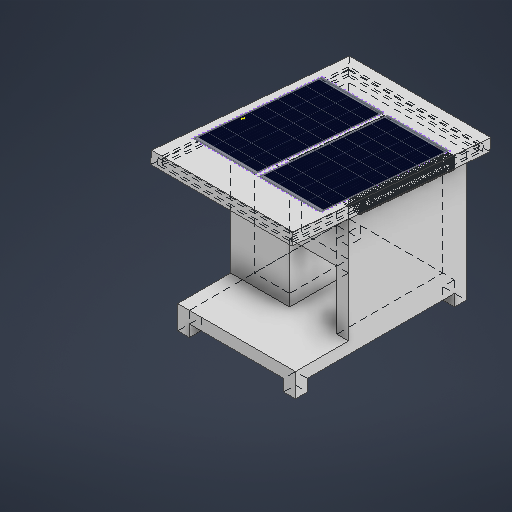
# Autodesk Inventor part: Cat House
Saved by Autodesk Inventor 2026 (Build 300175050, 175E)
## iProperties
Created: 2025-06-30
Part Number: Cat House
Material: Generic
Document SubType Name: Modeling
Designer: SWAT Loaner
Density: 1 g/cm^3
Appearance: Default
Author: SWAT Loaner
Autodesk Inventor part; units mm, degrees
ref_plane "YZ Plane" through (0, 0, 0) normal (1, 0, 0) x (0, 1, 0)
ref_plane "XZ Plane" through (0, 0, 0) normal (0, 1, 0) x (-1, 0, 0)
ref_plane "XY Plane" through (0, 0, 0) normal (0, 0, 1) x (1, 0, 0)
sketch "Sketch1" plane through (0, 0, 0) normal (1, 0, 0) x (0, 1, 0)
  line L0 (25.4, -25.4) -> (0, -25.4)
  line L1 (0, -25.4) -> (0, 0)
  line L2 (27.6222, 0) -> (28.9116, 14.7383)
  line L3 (25.4, -25.4) -> (25.1786, -27.9303)
  line L4 (28.9116, 14.7383) -> (31.442, 14.5169)
  line L5 (25.1786, -27.9303) -> (27.709, -28.1517)
  line L6 (27.709, -28.1517) -> (31.442, 14.5169)
  line L7 (27.6222, 0) -> (2.54, 0)
  line L8 (2.54, 0) -> (2.54, 11.43)
  line L9 (2.54, 11.43) -> (0, 11.43)
  line L10 (0, 11.43) -> (0, 0)
  dimension "d9" = 2.54
  dimension "d10" = 11.43
  constraints: 22 end point, 2 perpendicular, 1 horizontal, 1 point on line
  measures "d9" distance of L7.end L1.end
  measures "d10" distance of L7.end L8.end
extrude "Main Body" add sketch "Sketch1" along normal blind 25.4
sketch "Sketch2" plane through (25.4, 0, 0) normal (1, 0, 0) x (0, 0, -1)
  line L0 (-14.7383, 28.9116) -> (0, 27.6222) projected
  line L1 (-14.5169, 31.442) -> (-14.7383, 28.9116) projected
  line L2 (-14.7383, 28.9116) -> (-14.5169, 31.442)
  line L3 (27.9303, 25.1786) -> (28.1517, 27.709) projected
  line L4 (-14.5169, 31.442) -> (28.1517, 27.709)
  line L5 (25.4, 25.4) -> (27.9303, 25.1786) projected
  line L6 (28.1517, 27.709) -> (27.9303, 25.1786)
  line L7 (27.9303, 25.1786) -> (-14.7383, 28.9116)
  point P0 (0, 0)
  constraints: 8 end point, 2 collinear, 2 perpendicular
sketch "Sketch3" plane through (0, 0, 0) normal (-1, 0, 0) x (0, 0, 1)
  line L0 (-25.4, 25.4) -> (-27.9303, 25.1786) projected
  line L1 (-27.9303, 25.1786) -> (-28.1517, 27.709) projected
  line L2 (-27.9303, 25.1786) -> (-28.1517, 27.709)
  line L3 (14.5169, 31.442) -> (14.7383, 28.9116) projected
  line L4 (-28.1517, 27.709) -> (14.5169, 31.442)
  line L5 (14.7383, 28.9116) -> (0, 27.6222) projected
  line L6 (14.5169, 31.442) -> (14.7383, 28.9116)
  line L7 (14.7383, 28.9116) -> (-27.9303, 25.1786)
  point P0 (0, 0)
  constraints: 8 end point, 2 collinear, 2 perpendicular
extrude "Roof Extension 1" add sketch "Sketch3" along normal blind 2.54
extrude "Roof Extension 2" add sketch "Sketch2" along normal blind 2.54
sketch "Sketch4" plane through (0, 0, -25.4) normal (0, -1, 0) x (1, 0, 0)
  line L0 (25.4, 36.83) -> (25.4, 0) projected
  line L1 (25.4, 36.83) -> (22.86, 36.83)
  line L2 (22.86, 36.83) -> (22.86, 34.29)
  line L3 (22.86, 34.29) -> (25.4, 34.29)
  line L4 (25.4, 34.29) -> (25.4, 36.83)
  line L5 (22.86, 2.54) -> (22.86, 0)
  line L6 (22.86, 0) -> (25.4, 0)
  line L7 (25.4, 0) -> (25.4, 2.54)
  line L8 (25.4, 2.54) -> (22.86, 2.54)
  line L9 (0, 36.83) -> (0, 34.29)
  line L10 (0, 34.29) -> (2.54, 34.29)
  line L11 (2.54, 34.29) -> (2.54, 36.83)
  line L12 (2.54, 36.83) -> (0, 36.83)
  line L13 (0, 2.54) -> (0, 0)
  line L14 (0, 0) -> (2.54, 0)
  line L15 (2.54, 0) -> (2.54, 2.54)
  line L16 (2.54, 2.54) -> (0, 2.54)
  point P0 (0, 25.4)
  dimension "d17" = 2.54
  dimension "d18" = 2.54
  dimension "d21" = 34.29
  dimension "d24" = 22.86
  constraints: 32 end point, 2 horizontal, 2 parallel, 1 collinear, 1 perpendicular, 1 vertical, 23 other
  measures "d17" distance of L3.end L2.end
  measures "d18" distance of L2.end L1.end
  measures "d21" distance of L1.end L5.start
  measures "d24" distance of L1.end L9.start
extrude "Feet" add sketch "Sketch4" along normal blind 2.54
sketch "Sketch5" plane through (0, 2.54, 0) normal (0, 0, 1) x (1, 0, 0)
  line L0 (0, 0) -> (25.4, 0) projected
  line L1 (22.8718, 0) -> (12.7118, 0)
  line L2 (12.7118, 0) -> (12.7118, 12.7)
  line L3 (12.7118, 12.7) -> (22.8718, 12.7)
  line L4 (22.8718, 12.7) -> (22.8718, 0)
  point P0 (0, -2.54)
  point P1 (12.7118, 0)
  dimension "d29" = 10.16
  dimension "d30" = 12.7
  constraints: 8 end point, 2 parallel, 1 horizontal, 1 perpendicular, 1 point on line
  measures "d29" distance of L2.end L3.end
  measures "d30" distance of L1.end L2.end
shell "Shell" thickness 2.54 removed faces 0
extrude "Doorway 1" cut sketch "Sketch5" against normal blind 2.54
sketch "Sketch6" plane through (22.86, 27.4, -2.54) normal (0, 0, -1) x (-1, 0, 0)
  line L0 (10.1482, -12.16) -> (10.1482, -24.86) projected
  line L1 (10.1482, -24.86) -> (12.6882, -24.86)
  line L2 (12.6882, -24.86) -> (12.6882, 0.54)
  line L3 (12.6882, 0.54) -> (10.1482, 0.54)
  line L4 (10.1482, 0.54) -> (10.1482, -24.86)
  point P0 (22.86, -27.4)
  dimension "d34" = 2.54
  dimension "d35" = 25.4
  constraints: 8 end point, 2 parallel, 1 horizontal, 1 perpendicular
  measures "d34" distance of L3.end L2.end
  measures "d35" distance of L2.end L1.end
extrude "Inner Wall" add sketch "Sketch6" along normal up to surface (20.32 mm away)
sketch "Sketch7" plane through (12.7118, 2.54, 0) normal (1, 0, 0) x (0, 0, -1)
  line L0 (22.86, 23.0822) -> (22.86, 0) projected
  line L1 (22.86, 0) -> (12.7, 0)
  line L2 (12.7, 0) -> (12.7, 12.7)
  line L3 (12.7, 12.7) -> (22.86, 12.7)
  line L4 (22.86, 12.7) -> (22.86, 0)
  point P0 (0, -2.54)
  dimension "d38" = 10.16
  dimension "d39" = 12.7
  constraints: 8 end point, 2 parallel, 1 horizontal, 1 perpendicular
  measures "d38" distance of L2.end L3.end
  measures "d39" distance of L1.end L2.end
extrude "Doorway 2" cut sketch "Sketch7" against normal blind 2.54
sketch "Sketch8" plane through (25.4, 0, 0) normal (1, 0, 0) x (0, 0, -1)
  line L0 (2.54, 15.24) -> (2.54, 27.4) projected
  line L1 (22.86, 25.6222) -> (22.86, 15.24) projected
  line L2 (2.54, 27.4) -> (22.86, 25.6222)
  line L3 (22.86, 25.6222) -> (22.86, 23.0822)
  line L4 (22.86, 23.0822) -> (2.54, 24.86)
  line L5 (2.54, 27.4) -> (2.54, 24.86)
  line L6 (2.54, 24.86) -> (5.2799, 27.1603)
  line L7 (2.54, 24.86) -> (3.0461, 24.8157)
  line L8 (3.0461, 24.8157) -> (5.786, 27.116)
  line L9 (3.0461, 24.8157) -> (3.5521, 24.7714)
  line L10 (3.5521, 24.7714) -> (4.0582, 24.7272)
  line L11 (4.0582, 24.7272) -> (4.5643, 24.6829)
  line L12 (4.5643, 24.6829) -> (5.0703, 24.6386)
  line L13 (5.0703, 24.6386) -> (5.5764, 24.5943)
  line L14 (5.5764, 24.5943) -> (6.0825, 24.5501)
  line L15 (6.0825, 24.5501) -> (6.5885, 24.5058)
  line L16 (6.5885, 24.5058) -> (7.0946, 24.4615)
  line L17 (7.0946, 24.4615) -> (7.6007, 24.4172)
  line L18 (7.6007, 24.4172) -> (8.1067, 24.373)
  line L19 (8.1067, 24.373) -> (8.6128, 24.3287)
  line L20 (8.6128, 24.3287) -> (9.1189, 24.2844)
  line L21 (9.1189, 24.2844) -> (9.6249, 24.2401)
  line L22 (9.6249, 24.2401) -> (10.131, 24.1959)
  line L23 (10.131, 24.1959) -> (10.6371, 24.1516)
  line L24 (10.6371, 24.1516) -> (11.1431, 24.1073)
  line L25 (11.1431, 24.1073) -> (11.6492, 24.063)
  line L26 (11.6492, 24.063) -> (12.1553, 24.0188)
  line L27 (12.1553, 24.0188) -> (12.6613, 23.9745)
  line L28 (12.6613, 23.9745) -> (13.1674, 23.9302)
  line L29 (13.1674, 23.9302) -> (13.6735, 23.8859)
  line L30 (13.6735, 23.8859) -> (14.1795, 23.8417)
  line L31 (14.1795, 23.8417) -> (14.6856, 23.7974)
  line L32 (14.6856, 23.7974) -> (15.1917, 23.7531)
  line L33 (15.1917, 23.7531) -> (15.6977, 23.7088)
  line L34 (15.6977, 23.7088) -> (16.2038, 23.6646)
  line L35 (16.2038, 23.6646) -> (16.7099, 23.6203)
  line L36 (16.7099, 23.6203) -> (17.2159, 23.576)
  line L37 (17.2159, 23.576) -> (17.722, 23.5317)
  line L38 (17.722, 23.5317) -> (18.2281, 23.4875)
  line L39 (18.2281, 23.4875) -> (18.7341, 23.4432)
  line L40 (18.7341, 23.4432) -> (19.2402, 23.3989)
  line L41 (19.2402, 23.3989) -> (19.7463, 23.3546)
  line L42 (19.7463, 23.3546) -> (20.2523, 23.3104)
  line L43 (20.2523, 23.3104) -> (20.7584, 23.2661)
  line L44 (20.7584, 23.2661) -> (21.2645, 23.2218)
  line L45 (21.2645, 23.2218) -> (21.7705, 23.1775)
  line L46 (21.7705, 23.1775) -> (22.2766, 23.1333)
  line L47 (22.2766, 23.1333) -> (22.7827, 23.089)
  line L48 (3.5521, 24.7714) -> (6.2921, 27.0717)
  line L49 (4.5643, 24.6829) -> (7.3042, 26.9832)
  line L50 (5.0703, 24.6386) -> (7.8103, 26.9389)
  line L51 (4.0582, 24.7272) -> (6.7981, 27.0275)
  line L52 (5.5764, 24.5943) -> (8.3163, 26.8946)
  line L53 (6.0825, 24.5501) -> (8.8224, 26.8504)
  line L54 (6.5885, 24.5058) -> (9.3285, 26.8061)
  line L55 (7.0946, 24.4615) -> (9.8346, 26.7618)
  line L56 (7.6007, 24.4172) -> (10.3406, 26.7175)
  line L57 (8.1067, 24.373) -> (10.8467, 26.6733)
  line L58 (8.6128, 24.3287) -> (11.3528, 26.629)
  line L59 (9.1189, 24.2844) -> (11.8588, 26.5847)
  line L60 (9.6249, 24.2401) -> (12.3649, 26.5404)
  line L61 (10.131, 24.1959) -> (12.871, 26.4961)
  line L62 (10.6371, 24.1516) -> (13.377, 26.4519)
  line L63 (11.1431, 24.1073) -> (13.8831, 26.4076)
  line L64 (11.6492, 24.063) -> (14.3892, 26.3633)
  line L65 (12.1553, 24.0188) -> (14.8952, 26.319)
  line L66 (12.6613, 23.9745) -> (15.4013, 26.2748)
  line L67 (13.1674, 23.9302) -> (15.9074, 26.2305)
  line L68 (13.6735, 23.8859) -> (16.4134, 26.1862)
  line L69 (14.1795, 23.8417) -> (16.9195, 26.1419)
  line L70 (14.6856, 23.7974) -> (17.4256, 26.0977)
  line L71 (15.1917, 23.7531) -> (17.9316, 26.0534)
  line L72 (15.6977, 23.7088) -> (18.4377, 26.0091)
  line L73 (16.2038, 23.6646) -> (18.9438, 25.9648)
  line L74 (16.7099, 23.6203) -> (19.4498, 25.9206)
  line L75 (17.2159, 23.576) -> (19.9559, 25.8763)
  line L76 (17.722, 23.5317) -> (20.462, 25.832)
  line L77 (18.2281, 23.4875) -> (20.968, 25.7877)
  line L78 (18.7341, 23.4432) -> (21.4741, 25.7435)
  line L79 (19.2402, 23.3989) -> (21.9802, 25.6992)
  line L80 (19.7463, 23.3546) -> (22.4862, 25.6549)
  line L81 (20.2523, 23.3104) -> (22.86, 25.4996)
  line L82 (20.7584, 23.2661) -> (22.86, 25.0304)
  line L83 (21.2645, 23.2218) -> (22.86, 24.5613)
  line L84 (21.7705, 23.1775) -> (22.86, 24.0922)
  line L85 (22.2766, 23.1333) -> (22.86, 23.623)
  line L86 (2.54, 27.2057) -> (2.7496, 27.3817)
  line L87 (2.54, 26.7365) -> (3.2557, 27.3374)
  line L88 (2.54, 25.7983) -> (4.2678, 27.2488)
  line L89 (2.54, 25.3291) -> (4.7739, 27.2046)
  line L90 (2.54, 26.2674) -> (3.7617, 27.2931)
  line L91 (2.54, 24.86) -> (5.2799, 27.1603)
  line L92 (2.793, 24.8379) -> (5.533, 27.1381)
  line L93 (3.2991, 24.7936) -> (6.039, 27.0939)
  line L94 (3.8052, 24.7493) -> (6.5451, 27.0496)
  line L95 (4.8173, 24.6608) -> (7.5572, 26.961)
  line L96 (5.3234, 24.6165) -> (8.0633, 26.9168)
  line L97 (4.3112, 24.705) -> (7.0512, 27.0053)
  line L98 (5.8294, 24.5722) -> (8.5694, 26.8725)
  line L99 (6.3355, 24.5279) -> (9.0755, 26.8282)
  line L100 (6.8416, 24.4837) -> (9.5815, 26.7839)
  line L101 (7.3476, 24.4394) -> (10.0876, 26.7397)
  line L102 (7.8537, 24.3951) -> (10.5937, 26.6954)
  line L103 (8.3598, 24.3508) -> (11.0997, 26.6511)
  line L104 (8.8658, 24.3066) -> (11.6058, 26.6068)
  line L105 (9.3719, 24.2623) -> (12.1119, 26.5626)
  line L106 (9.878, 24.218) -> (12.6179, 26.5183)
  line L107 (10.384, 24.1737) -> (13.124, 26.474)
  line L108 (10.8901, 24.1295) -> (13.6301, 26.4297)
  line L109 (11.3962, 24.0852) -> (14.1361, 26.3855)
  line L110 (11.9022, 24.0409) -> (14.6422, 26.3412)
  line L111 (12.4083, 23.9966) -> (15.1483, 26.2969)
  line L112 (12.9144, 23.9524) -> (15.6543, 26.2526)
  line L113 (13.4204, 23.9081) -> (16.1604, 26.2084)
  line L114 (13.9265, 23.8638) -> (16.6665, 26.1641)
  line L115 (14.4326, 23.8195) -> (17.1725, 26.1198)
  line L116 (14.9386, 23.7753) -> (17.6786, 26.0755)
  line L117 (15.4447, 23.731) -> (18.1847, 26.0313)
  line L118 (15.9508, 23.6867) -> (18.6907, 25.987)
  line L119 (16.4568, 23.6424) -> (19.1968, 25.9427)
  line L120 (16.9629, 23.5982) -> (19.7029, 25.8984)
  line L121 (17.469, 23.5539) -> (20.2089, 25.8542)
  line L122 (17.975, 23.5096) -> (20.715, 25.8099)
  line L123 (18.4811, 23.4653) -> (21.2211, 25.7656)
  line L124 (18.9872, 23.421) -> (21.7271, 25.7213)
  line L125 (19.4932, 23.3768) -> (22.2332, 25.6771)
  line L126 (19.9993, 23.3325) -> (22.7393, 25.6328)
  line L127 (20.5054, 23.2882) -> (22.86, 25.265)
  line L128 (21.0114, 23.2439) -> (22.86, 24.7959)
  line L129 (21.5175, 23.1997) -> (22.86, 24.3267)
  line L130 (22.0236, 23.1554) -> (22.86, 23.8576)
  line L131 (22.5296, 23.1111) -> (22.86, 23.3885)
  line L132 (2.54, 26.9711) -> (3.0026, 27.3595)
  line L133 (2.54, 26.502) -> (3.5087, 27.3152)
  line L134 (2.54, 26.0328) -> (4.0148, 27.271)
  line L135 (2.54, 25.5637) -> (4.5208, 27.2267)
  line L136 (2.54, 25.0946) -> (5.0269, 27.1824)
  point P0 (0, 0)
  dimension "d42" = 2.54
  dimension "d44" = 0.508
  dimension "d45" = 0.508
  dimension "d46" = 0.508
  dimension "d47" = 0.508
  dimension "d48" = 0.508
  dimension "d49" = 0.508
  dimension "d50" = 0.508
  dimension "d51" = 0.508
  dimension "d52" = 0.508
  dimension "d53" = 0.508
  dimension "d54" = 0.508
  dimension "d55" = 0.508
  dimension "d56" = 0.508
  dimension "d57" = 0.508
  dimension "d58" = 0.508
  dimension "d59" = 0.508
  dimension "d60" = 0.508
  dimension "d61" = 0.508
  dimension "d62" = 0.508
  dimension "d63" = 0.508
  dimension "d64" = 0.508
  dimension "d65" = 0.508
  dimension "d66" = 0.508
  dimension "d67" = 0.508
  dimension "d68" = 0.508
  dimension "d69" = 0.508
  dimension "d70" = 0.508
  dimension "d71" = 0.508
  dimension "d72" = 0.508
  dimension "d73" = 0.508
  dimension "d74" = 0.508
  dimension "d75" = 0.508
  dimension "d76" = 0.508
  dimension "d77" = 0.508
  dimension "d78" = 0.508
  dimension "d79" = 0.508
  dimension "d80" = 0.508
  dimension "d81" = 0.508
  dimension "d82" = 0.508
  dimension "d83" = 0.508
  dimension "d90" = 0.508
  dimension "d91" = 0.508
  dimension "d92" = 0.508
  dimension "d93" = 0.508
  dimension "d94" = 0.508
  dimension "d95" = 0.508
  dimension "d96" = 0.508
  dimension "d97" = 0.508
  dimension "d98" = 0.508
  dimension "d99" = 0.508
  dimension "d100" = 0.508
  dimension "d101" = 0.508
  dimension "d102" = 0.508
  dimension "d103" = 0.508
  dimension "d104" = 0.508
  dimension "d105" = 0.508
  dimension "d106" = 0.508
  dimension "d107" = 0.508
  dimension "d108" = 0.508
  dimension "d109" = 0.508
  dimension "d110" = 0.508
  dimension "d111" = 0.508
  dimension "d112" = 0.508
  constraints: 266 end point, 88 parallel, 10 point on line, 76 other
  measures "d42" distance of L3.start L3.end
  measures "d44" distance of L5.end L7.end
  measures "d45" distance of L7.end L9.end
  measures "d46" distance of L9.end L10.end
  measures "d47" distance of L10.end L11.end
  measures "d48" distance of L11.end L12.end
  measures "d49" distance of L12.end L13.end
  measures "d50" distance of L13.end L14.end
  measures "d51" distance of L14.end L15.end
  measures "d52" distance of L15.end L16.end
  measures "d53" distance of L16.end L17.end
  measures "d54" distance of L17.end L18.end
  measures "d55" distance of L18.end L19.end
  measures "d56" distance of L19.end L20.end
  measures "d57" distance of L20.end L21.end
  measures "d58" distance of L21.end L22.end
  measures "d59" distance of L22.end L23.end
  measures "d60" distance of L23.end L24.end
  measures "d61" distance of L24.end L25.end
  measures "d62" distance of L25.end L26.end
  measures "d63" distance of L26.end L27.end
  measures "d64" distance of L27.end L28.end
  measures "d65" distance of L28.end L29.end
  measures "d66" distance of L29.end L30.end
  measures "d67" distance of L30.end L31.end
  measures "d68" distance of L31.end L32.end
  measures "d69" distance of L32.end L33.end
  measures "d70" distance of L33.end L34.end
  measures "d71" distance of L34.end L35.end
  measures "d72" distance of L35.end L36.end
  measures "d73" distance of L36.end L37.end
  measures "d74" distance of L37.end L38.end
  measures "d75" distance of L38.end L39.end
  measures "d76" distance of L39.end L40.end
  measures "d77" distance of L40.end L41.end
  measures "d78" distance of L41.end L42.end
  measures "d79" distance of L42.end L43.end
  measures "d80" distance of L43.end L44.end
  measures "d81" distance of L44.end L45.end
  measures "d82" distance of L45.end L46.end
  measures "d83" distance of L46.end L47.end
  measures "d90" distance of L92.start L93.start
  measures "d91" distance of L93.start L94.start
  measures "d92" distance of L94.start L97.start
  measures "d93" distance of L97.start L95.start
  measures "d94" distance of L95.start L96.start
  measures "d95" distance of L96.start L98.start
  measures "d96" distance of L98.start L99.start
  measures "d97" distance of L99.start L100.start
  measures "d98" distance of L100.start L101.start
  measures "d99" distance of L101.start L102.start
  measures "d100" distance of L102.start L103.start
  measures "d101" distance of L103.start L104.start
  measures "d102" distance of L104.start L105.start
  measures "d103" distance of L105.start L106.start
  measures "d104" distance of L106.start L107.start
  measures "d105" distance of L107.start L108.start
  measures "d106" distance of L108.start L109.start
  measures "d107" distance of L109.start L110.start
  measures "d108" distance of L110.start L111.start
  measures "d109" distance of L111.start L112.start
  measures "d110" distance of L112.start L113.start
  measures "d111" distance of L113.start L114.start
  measures "d112" distance of L114.start L115.start
extrude "Ventillation" cut sketch "Sketch8" against normal through all contours L0 L136 L2 L6 | L92 L2 L8 L4 | L0 L135 L2 L89 | L93 L2 L48 L4 | L0 L134 L2 L88 | L94 L2 L51 L4 | L0 L133 L2 L90 | L97 L2 L49 L4 | L0 L132 L2 L87 | L95 L2 L50 L4 | L0 L2 L86 | L96 L2 L52 L4 | L98 L2 L53 L4 | L99 L2 L54 L4 | L100 L2 L55 L4 | L101 L2 L56 L4 | L102 L2 L57 L4 | L103 L2 L58 L4 | L104 L2 L59 L4 | L105 L2 L60 L4 | L106 L2 L61 L4 | L107 L2 L62 L4 | L108 L2 L63 L4 | L109 L2 L64 L4 | L110 L2 L65 L4 | L111 L2 L66 L4 | L112 L2 L67 L4 | L113 L2 L68 L4 | L114 L2 L69 L4 | L115 L2 L70 L4 | L116 L2 L71 L4 | L117 L2 L72 L4 | L118 L2 L73 L4 | L119 L2 L74 L4 | L120 L2 L75 L4 | L121 L2 L76 L4 | L122 L2 L77 L4 | L123 L2 L78 L4 | L124 L2 L79 L4 | L125 L2 L80 L4 | L126 L2 L1 L81 L4 | L127 L1 L82 L4 | L128 L1 L83 L4 | L129 L1 L84 L4 | L130 L1 L85 L4 | L131 L1 L4
sketch "Sketch9" plane through (-2.54, 25.1786, -27.9303) normal (0, -0.9961947, 0.0871557) x (1, 0, 0)
  line L0 (0, 42.8316) -> (30.48, 42.8316)
  line L1 (30.48, 42.8316) -> (30.48, 0)
  line L2 (30.48, 0) -> (0, 0)
  line L3 (0, 0) -> (0, 42.8316)
  line L4 (29.21, 41.5616) -> (1.27, 41.5616)
  line L5 (1.27, 41.5616) -> (1.27, 1.27)
  line L6 (1.27, 1.27) -> (29.21, 1.27)
  line L7 (29.21, 1.27) -> (29.21, 41.5616)
  line L8 (0.762, 42.0696) -> (29.718, 42.0696)
  line L9 (29.718, 42.0696) -> (29.718, 0.762)
  line L10 (29.718, 0.762) -> (0.762, 0.762)
  line L11 (0.762, 0.762) -> (0.762, 42.0696)
  point P0 (2.54, 25.6296)
  dimension "d131" = 1.27
  dimension "d132" = 0.508
  constraints: 24 end point, 6 parallel, 3 perpendicular, 1 horizontal, 6 other
  measures "d131" distance between parallel lines of L0 L4
  measures "d132" distance between parallel lines of L4 L8
extrude "LED Strip" cut sketch "Sketch9" against normal blind 1.27 contours L8 L9 L10 L11
sketch "Solar Panels" plane through (-2.54, 31.442, 14.5169) normal (0, 0.9961947, -0.0871557) x (1, 0, 0)
  line L0 (1.4309, 35.4226) -> (15.0978, 35.4226) construction
  line L1 (15.0978, 35.4226) -> (15.0978, 7.1926) construction
  line L2 (15.0978, 7.1926) -> (1.4309, 7.1926) construction
  line L3 (1.4309, 7.1926) -> (1.4309, 35.4226) construction
  line L4 (15.6265, 35.3696) -> (29.2934, 35.3696) construction
  line L5 (29.2934, 35.3696) -> (29.2934, 7.1396) construction
  line L6 (29.2934, 7.1396) -> (15.6265, 7.1396) construction
  line L7 (15.6265, 7.1396) -> (15.6265, 35.3696) construction
  point P0 (2.54, 17.202)
  constraints: 4 other
body "Solid1"
